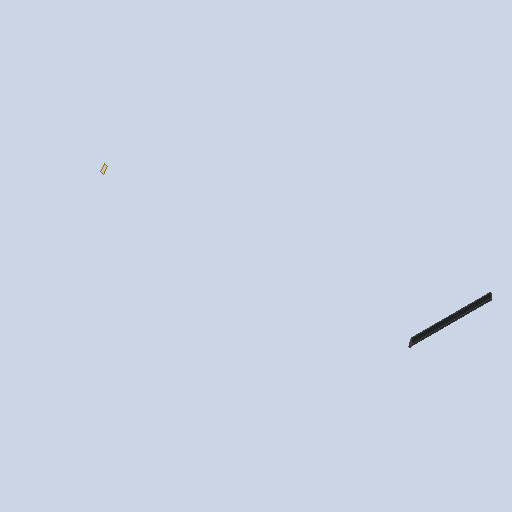
# Autodesk Inventor part: LeftAlerion
Saved by Autodesk Inventor 2025.2 (Build 292293000, 293)
## iProperties
Created: 2025-03-16
Part Number: LeftAlerion
Material: Generic
Document SubType Name: Modeling
Designer: Cupri
Density: 1 g/cm^3
Appearance: Default
Author: Cupri
Autodesk Inventor part; units mm, degrees
ref_plane "YZ Plane" through (0, 0, 0) normal (1, 0, 0) x (0, 1, 0)
ref_plane "XZ Plane" through (0, 0, 0) normal (0, 1, 0) x (-1, 0, 0)
ref_plane "Work Plane1" through (-2925.2733, -622.4324, 0) normal (0, 0, 1) x (0.9219818, -0.3872333, 0)
sketch "Sketch1" plane through (-2925.2733, -622.4324, 0) normal (0, 0, 1) x (0.9219818, -0.3872333, 0)
  line L0 (2457.337, 1676.7645) -> (2462.4983, 1678.9322) projected
  line L1 (2446.8172, 1741.2195) -> (2445.9191, 1740.8423) projected
  spline S0 degree 3 poles (2445.9191, 1740.8423) (2446.3533, 1738.0048) (2446.4804, 1737.1605) (2447.5243, 1730.1637) (2447.849, 1727.9846) (2448.2125, 1725.6073) knots -1.334504 -1.334504 -1.334504 -1.334504 -0.473358 -0.473358 0 0 0 0 projected
  line L2 (2473.5621, 1683.579) -> (2476.43, 1684.7835) projected
  circle A0 centre (1.2437, -14.4504) radius 2 projected
  circle A1 centre (1.2437, -14.4504) radius 1 projected
  circle A2 centre (1.2437, -14.4504) radius 2
  line L3 (2464.4236, 1705.3371) -> (2473.5621, 1683.579) projected
  line L4 (2476.43, 1684.7835) -> (2473.5621, 1683.579) projected
  spline S1 degree 3 poles (2446.8172, 1741.2195) (2451.7124, 1732.0048) (2452.4978, 1730.4494) (2465.2393, 1706.1586) (2470.4628, 1696.2474) (2476.43, 1684.7835) knots -8.256346 -8.256346 -8.256346 -8.256346 -3.940963 -3.940963 -0.050257 -0.050257 -0.050257 -0.050257 projected
  line L5 (2445.9191, 1740.8423) -> (2446.8172, 1741.2195) projected
  spline S2 degree 3 poles (2448.2125, 1725.6073) (2447.849, 1727.9846) (2447.5243, 1730.1637) (2446.4804, 1737.1605) (2446.3533, 1738.0048) (2445.9191, 1740.8423) knots -1.334504 -1.334504 -1.334504 -1.334504 -0.861145 -0.861145 0 0 0 0 projected
  spline S3 degree 3 poles (2457.337, 1676.7645) (2455.4989, 1685.3573) (2453.6106, 1694.6448) (2450.5029, 1711.682) (2449.0652, 1720.1585) (2448.2125, 1725.6073) knots -3.742267 -3.742267 -3.742267 -3.742267 -1.654546 -1.654546 0 0 0 0 projected
  line L6 (2462.4983, 1678.9322) -> (2457.337, 1676.7645) projected
  line L7 (2462.4983, 1678.9322) -> (2453.3598, 1700.6903) projected
  line L8 (2453.3598, 1700.6903) -> (2464.4236, 1705.3371) projected
  circle A3 centre (-81.1133, -14.9806) radius 1
  line L9 (2457.337, 1676.7645) -> (2476.43, 1684.7835)
  arc A4 (2457.337, 1676.7645) -> (2464.3672, 1707.8287) centre (2449.7591, 1694.807) ccw
  line L10 (2453.3598, 1700.6903) -> (2464.4236, 1705.3371) projected
  line L11 (2464.4236, 1705.3371) -> (2473.5621, 1683.579) projected
  line L12 (2462.4983, 1678.9322) -> (2453.3598, 1700.6903) projected
  spline S4 degree 3 poles (2476.43, 1684.7835) (2470.4628, 1696.2474) (2465.2393, 1706.1586) (2452.4978, 1730.4494) (2451.7124, 1732.0048) (2446.8172, 1741.2195) knots -8.256346 -8.256346 -8.256346 -8.256346 -4.36564 -4.36564 -0.050257 -0.050257 -0.050257 -0.050257 projected
  spline S5 degree 3 poles (2448.2125, 1725.6073) (2449.0652, 1720.1585) (2450.5029, 1711.682) (2453.6106, 1694.6448) (2455.4989, 1685.3573) (2457.337, 1676.7645) knots -3.742267 -3.742267 -3.742267 -3.742267 -2.087721 -2.087721 0 0 0 0 projected
  point P0 (2456.022, 1706.6346)
  constraints: 3 centre point, 2 end point, 2 point on circle, 1 coincident, 1 concentric, 1 tangent, 4 other
ref_plane "Work Plane2" through (-21.4445, -212.198, 623.3738) normal (0, 0.0865745, 0.9962454) x (1, 0, 0)
extrude "Extrusion1" add sketch "Sketch1" along normal up to surface contours S3 S0 L1 S1 A4 L3 L8 L7 | L7 L8 L3 A4 | S1 A4 surface through (-21.4445, -212.198, 623.3738) normal (0, 0.0865745, 0.9962454)
body "Solid1"
